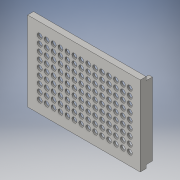
# Autodesk Inventor part: RaspPiCaseTop
Saved by Autodesk Inventor 2016 (Build 200138000, 138)
## iProperties
Created: 2016-04-29
Part Number: RaspPiCaseTop
Material: Generic
Document SubType Name: Modeling
Designer: mkepler
Density: 1 g/cm^3
Appearance: Default
Author: mkepler
Autodesk Inventor part; units mm, degrees
ref_plane "YZ Plane" through (0, 0, 0) normal (1, 0, 0) x (0, 1, 0)
ref_plane "XZ Plane" through (0, 0, 0) normal (0, 1, 0) x (-1, 0, 0)
ref_plane "XY Plane" through (0, 0, 0) normal (0, 0, 1) x (1, 0, 0)
sketch "Sketch1" plane through (0, 0, 0) normal (0, 1, 0) x (-1, 0, 0)
  line L0 (0, 0) -> (91.5, 0)
  line L1 (91.5, 0) -> (91.5, -63)
  line L2 (91.5, -63) -> (0, -63)
  circle A0 centre (84, -7.5) radius 2.15
  circle A1 centre (84, -13.5) radius 2.15
  circle A2 centre (84, -19.5) radius 2.15
  circle A3 centre (84, -25.5) radius 2.15
  circle A4 centre (84, -31.5) radius 2.15
  circle A5 centre (84, -55.5) radius 2.15
  circle A6 centre (84, -49.5) radius 2.15
  circle A7 centre (84, -43.5) radius 2.15
  circle A8 centre (84, -37.5) radius 2.15
  circle A9 centre (78, -7.5) radius 2.15
  circle A10 centre (78, -13.5) radius 2.15
  circle A11 centre (78, -19.5) radius 2.15
  circle A12 centre (78, -25.5) radius 2.15
  circle A13 centre (78, -31.5) radius 2.15
  circle A14 centre (78, -37.5) radius 2.15
  circle A15 centre (78, -43.5) radius 2.15
  circle A16 centre (78, -49.5) radius 2.15
  circle A17 centre (78, -55.5) radius 2.15
  circle A18 centre (66, -7.5) radius 2.15
  circle A19 centre (66, -13.5) radius 2.15
  circle A20 centre (66, -19.5) radius 2.15
  circle A21 centre (66, -25.5) radius 2.15
  circle A22 centre (66, -31.5) radius 2.15
  circle A23 centre (66, -37.5) radius 2.15
  circle A24 centre (66, -43.5) radius 2.15
  circle A25 centre (66, -49.5) radius 2.15
  circle A26 centre (66, -55.5) radius 2.15
  circle A27 centre (72, -37.5) radius 2.15
  circle A28 centre (72, -31.5) radius 2.15
  circle A29 centre (72, -25.5) radius 2.15
  circle A30 centre (72, -19.5) radius 2.15
  circle A31 centre (72, -13.5) radius 2.15
  circle A32 centre (72, -7.5) radius 2.15
  circle A33 centre (72, -49.5) radius 2.15
  circle A34 centre (72, -55.5) radius 2.15
  circle A35 centre (72, -43.5) radius 2.15
  line L3 (66, -55.5) -> (63, -55.5)
  line L4 (63, -55.5) -> (63, -45.305)
  circle A36 centre (42, -7.5) radius 2.15
  circle A37 centre (42, -13.5) radius 2.15
  circle A38 centre (42, -19.5) radius 2.15
  circle A39 centre (42, -25.5) radius 2.15
  circle A40 centre (42, -31.5) radius 2.15
  circle A41 centre (42, -37.5) radius 2.15
  circle A42 centre (42, -43.5) radius 2.15
  circle A43 centre (42, -49.5) radius 2.15
  circle A44 centre (42, -55.5) radius 2.15
  circle A45 centre (48, -37.5) radius 2.15
  circle A46 centre (48, -31.5) radius 2.15
  circle A47 centre (48, -25.5) radius 2.15
  circle A48 centre (48, -19.5) radius 2.15
  circle A49 centre (48, -13.5) radius 2.15
  circle A50 centre (48, -7.5) radius 2.15
  circle A51 centre (48, -49.5) radius 2.15
  circle A52 centre (48, -55.5) radius 2.15
  circle A53 centre (48, -43.5) radius 2.15
  circle A54 centre (60, -37.5) radius 2.15
  circle A55 centre (54, -37.5) radius 2.15
  circle A56 centre (60, -31.5) radius 2.15
  circle A57 centre (54, -31.5) radius 2.15
  circle A58 centre (60, -25.5) radius 2.15
  circle A59 centre (54, -25.5) radius 2.15
  circle A60 centre (60, -19.5) radius 2.15
  circle A61 centre (60, -13.5) radius 2.15
  circle A62 centre (54, -13.5) radius 2.15
  circle A63 centre (54, -7.5) radius 2.15
  circle A64 centre (54, -19.5) radius 2.15
  circle A65 centre (60, -7.5) radius 2.15
  circle A66 centre (60, -43.5) radius 2.15
  circle A67 centre (54, -43.5) radius 2.15
  circle A68 centre (54, -49.5) radius 2.15
  circle A69 centre (54, -55.5) radius 2.15
  circle A70 centre (60, -55.5) radius 2.15
  circle A71 centre (60, -49.5) radius 2.15
  line L5 (42, -55.5) -> (39, -55.5)
  line L6 (39, -55.5) -> (39, -51.65)
  circle A72 centre (12, -37.5) radius 2.15
  circle A73 centre (6, -37.5) radius 2.15
  circle A74 centre (12, -31.5) radius 2.15
  circle A75 centre (6, -31.5) radius 2.15
  circle A76 centre (12, -25.5) radius 2.15
  circle A77 centre (6, -25.5) radius 2.15
  circle A78 centre (12, -19.5) radius 2.15
  circle A79 centre (12, -13.5) radius 2.15
  circle A80 centre (6, -13.5) radius 2.15
  circle A81 centre (6, -7.5) radius 2.15
  circle A82 centre (6, -19.5) radius 2.15
  circle A83 centre (12, -7.5) radius 2.15
  circle A84 centre (12, -43.5) radius 2.15
  circle A85 centre (6, -43.5) radius 2.15
  circle A86 centre (6, -49.5) radius 2.15
  circle A87 centre (6, -55.5) radius 2.15
  circle A88 centre (12, -55.5) radius 2.15
  circle A89 centre (12, -49.5) radius 2.15
  line L7 (12, -55.5) -> (15, -55.5)
  line L8 (15, -55.5) -> (15, -45.305)
  circle A90 centre (36, -49.5) radius 2.15
  circle A91 centre (36, -43.5) radius 2.15
  circle A92 centre (30, -55.5) radius 2.15
  circle A93 centre (30, -49.5) radius 2.15
  circle A94 centre (30, -43.5) radius 2.15
  circle A95 centre (24, -55.5) radius 2.15
  circle A96 centre (24, -49.5) radius 2.15
  circle A97 centre (24, -43.5) radius 2.15
  circle A98 centre (36, -55.5) radius 2.15
  circle A99 centre (36, -37.5) radius 2.15
  circle A100 centre (36, -7.5) radius 2.15
  circle A101 centre (36, -13.5) radius 2.15
  circle A102 centre (30, -25.5) radius 2.15
  circle A103 centre (30, -19.5) radius 2.15
  circle A104 centre (30, -13.5) radius 2.15
  circle A105 centre (30, -7.5) radius 2.15
  circle A106 centre (18, -25.5) radius 2.15
  circle A107 centre (24, -25.5) radius 2.15
  circle A108 centre (18, -19.5) radius 2.15
  circle A109 centre (24, -19.5) radius 2.15
  circle A110 centre (18, -13.5) radius 2.15
  circle A111 centre (24, -13.5) radius 2.15
  circle A112 centre (24, -7.5) radius 2.15
  circle A113 centre (18, -7.5) radius 2.15
  circle A114 centre (36, -19.5) radius 2.15
  circle A115 centre (36, -25.5) radius 2.15
  circle A116 centre (36, -31.5) radius 2.15
  circle A117 centre (30, -37.5) radius 2.15
  circle A118 centre (24, -37.5) radius 2.15
  circle A119 centre (24, -31.5) radius 2.15
  circle A120 centre (30, -31.5) radius 2.15
  circle A121 centre (18, -49.5) radius 2.15
  circle A122 centre (18, -43.5) radius 2.15
  circle A123 centre (18, -55.5) radius 2.15
  circle A124 centre (18, -37.5) radius 2.15
  circle A125 centre (18, -31.5) radius 2.15
  line L9 (36, -55.5) -> (39, -55.5)
  line L10 (0, 0) -> (0, -63)
  dimension "d0" = 91.5
  dimension "d1" = 63
  dimension "d2" = 4.3
  dimension "d3" = 7.5
  dimension "d4" = 7.5
  dimension "d5" = 4.3
  dimension "d6" = 6
  dimension "d7" = 4.3
  dimension "d8" = 6
  dimension "d9" = 4.3
  dimension "d10" = 6
  dimension "d11" = 4.3
  dimension "d12" = 6
  dimension "d15" = 6
  dimension "d17" = 3
  dimension "d18" = 3
  constraints: 126 centre point, 92 symmetric about line, 22 end point, 3 horizontal, 3 perpendicular, 1 parallel, 1 vertical, 90 other
  measures "d0" distance of L1.end L2.end
  measures "d1" distance of L0.end L1.end
  measures "d2" diameter of A0
  measures "d3" distance from line of L0 A0.centre
  measures "d4" distance from line of L1 A0.centre
  measures "d5" diameter of A1
  measures "d6" distance of A1.centre A0.centre
  measures "d7" diameter of A2
  measures "d8" distance of A1.centre A2.centre
  measures "d9" diameter of A3
  measures "d10" distance of A2.centre A3.centre
  measures "d11" diameter of A4
  measures "d12" distance of A3.centre A4.centre
  measures "d15" distance of A17.centre A5.centre
  measures "d17" distance of L3.start L3.end
  measures "d18" distance of L5.start L5.end
extrude "Extrusion1" add sketch "Sketch1" along normal blind 1.5
sketch "Sketch2" plane through (0, 1.5, 0) normal (0, 1, 0) x (1, 0, 0)
  line L0 (3, 0) -> (3, -3)
  line L1 (3, -3) -> (-94.5, -3)
  line L2 (-94.5, -3) -> (-94.5, 66)
  line L3 (-94.5, 66) -> (3, 66)
  line L4 (3, 66) -> (3, 0)
  line L5 (-91.5, 63) -> (-91.5, 0) projected
  line L6 (0, 63) -> (-91.5, 63) projected
  line L7 (-91.5, 0) -> (0, 0)
  line L8 (0, 0) -> (0, 63)
  line L9 (0, 63) -> (-91.5, 63)
  line L10 (-91.5, 63) -> (-91.5, 0)
  dimension "d30" = 97.5
  dimension "d31" = 69
  dimension "d32" = 97.5
  constraints: 18 end point, 3 perpendicular, 2 parallel, 1 horizontal, 1 vertical
  measures "d30" distance of L0.end L1.end
  measures "d31" distance of L1.end L2.end
  measures "d32" distance of L2.end L3.end
extrude "Extrusion2" add sketch "Sketch2" along normal blind 3.612 and the other way blind 1.5
sketch "Sketch5" plane through (0, 1.5, 0) normal (0, 1, 0) x (1, 0, 0)
  point P0 (0, 0)
sketch "Sketch6" plane through (0, 5.112, 0) normal (0, 1, 0) x (1, 0, 0)
  line L0 (0, 0) -> (0, 63) projected
  line L1 (3, 66) -> (3, -3) projected
  line L2 (0, 0) -> (3, 0)
  line L3 (3, 0) -> (3, 63)
  line L4 (3, 63) -> (0, 63)
  line L5 (0, 63) -> (0, 0)
  constraints: 8 end point, 2 parallel, 1 horizontal, 1 perpendicular, 1 point on line
extrude "Extrusion3" add sketch "Sketch6" along normal blind 5.388
body "Solid1"
